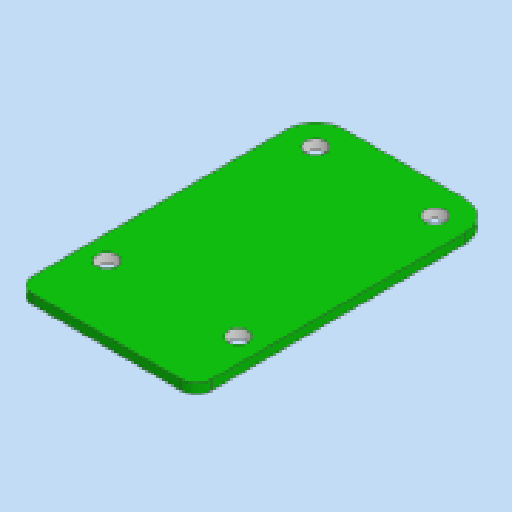
# Autodesk Inventor part: mcu_pcb
Saved by Autodesk Inventor 2024 (Build 280153000, 153)
## iProperties
Created: 2025-05-06
Part Number: mcu_pcb
Material: Generic
Document SubType Name: Modeling
Designer: XxPan
Density: 1 g/cm^3
Appearance: Default
Author: XxPan
Autodesk Inventor part; units mm, degrees
ref_plane "YZ Plane" through (0, 0, 0) normal (1, 0, 0) x (0, 1, 0)
ref_plane "XZ Plane" through (0, 0, 0) normal (0, 1, 0) x (-1, 0, 0)
ref_plane "XY Plane" through (0, 0, 0) normal (0, 0, 1) x (1, 0, 0)
sketch "Sketch1" plane through (0, 0, 0) normal (0, 1, 0) x (-1, 0, 0)
  line L0 (15, 25) -> (-15, 25)
  line L1 (-15, 25) -> (-15, -25)
  line L2 (-15, -25) -> (15, -25)
  line L3 (15, -25) -> (15, 25)
  line L4 (21, 0) -> (-21, 0) construction
  line L5 (0, -35) -> (0, 35) construction
  point P0 (0, 0)
  dimension "d11" = 15
  dimension "d12" = 15
  dimension "d13" = 25
  dimension "d14" = 25
  constraints: 8 end point, 2 parallel, 1 horizontal, 1 perpendicular
  measures "d11" distance between parallel lines of L1 L5
  measures "d12" distance between parallel lines of L5 L3
  measures "d13" distance between parallel lines of L4 L0
  measures "d14" distance between parallel lines of L4 L2
extrude "Extrusion1" add sketch "Sketch1" along normal blind 1.6
fillet "Fillet1" radius 2.5 2 edges at (-15, 0.8, 25) (15, 0.8, 25)
fillet "Fillet2" radius 5 2 edges at (-15, 0.8, -25) (15, 0.8, -25)
sketch "Sketch3" plane through (0, 0, 0) normal (0, -1, 0) x (1, 0, 0)
  arc A0 (10, -25) -> (15, -20) centre (10, -20) ccw projected
  arc A1 (-15, -20) -> (-10, -25) centre (-10, -20) ccw projected
  line L0 (15, 22.5) -> (15, -20) projected
  line L1 (-15, -20) -> (-15, 22.5) projected
  line L2 (-12.5, 25) -> (12.5, 25) projected
  point P0 (0, 0)
  point P1 (11, 14)
  point P2 (-11, 14)
  dimension "d24" = 4
  dimension "d25" = 4
  dimension "d26" = 11
  constraints: 2 coincident, 1 horizontal alignment
  measures "d24" distance from line of L0 point (11, 14)
  measures "d25" distance from line of L1 point (-11, 14)
  measures "d26" distance from line of point (11, 14) L2
hole "Hole2" at (10, 0, -20) at (-10, 0, -20) at (11, 0, 14) at (-11, 0, 14) direction (0, 1, 0) diameter 3.4 end through all
body "Solid1"
